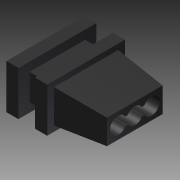
# Autodesk Inventor part: 276-2154
Saved by Autodesk Inventor 2013 (Build 170138000, 138)
## iProperties
Category: Sensors
Company: Autodesk Inc.
Created: 2012-03-30
Part Number: 276-2154
Document SubType Name: Modeling
Designer: Autodesk Inc.
Density: 0.93 g/cm^3
Material: Rubber
Catalog Web Link: http://www.vexrobotics.com/276-2154.html
Vendor: VEX
Mass: 0.0908272 g
Surface Area: 3.07194 cm^2
Volume: 0.0976637 cm^3
Author: Autodesk Inc.
Autodesk Inventor part; units mm, degrees
ref_plane "YZ Plane" through (0, 0, 0) normal (1, 0, 0) x (0, 1, 0)
ref_plane "XZ Plane" through (0, 0, 0) normal (0, 1, 0) x (-1, 0, 0)
ref_plane "XY Plane" through (0, 0, 0) normal (0, 0, 1) x (1, 0, 0)
sketch "Sketch1" plane through (0, 0, 0) normal (0, 0, 1) x (1, 0, 0)
  line L0 (0, 0) -> (7.0104, 0)
  line L1 (7.0104, 0) -> (7.0104, 3.9878)
  line L2 (7.0104, 3.9878) -> (0, 3.9878)
  line L3 (0, 3.9878) -> (0, 0)
  dimension "d0" = 7.0104
  dimension "d1" = 3.9878
  constraints: 8 end point, 2 parallel, 1 horizontal, 1 perpendicular
  measures "d0" distance of L2.end L1.end
  measures "d1" distance of L1.end L0.end
extrude "Extrusion1" add sketch "Sketch1" against normal blind 1.0922
sketch "Sketch2" plane through (0, 0, -1.0922) normal (0, 0, -1) x (-1, 0, 0)
  line L0 (-7.0104, 0) -> (-7.0104, 3.9878) projected
  line L1 (-7.0104, 3.9878) -> (0, 3.9878) projected
  line L2 (-6.0071, 0.8001) -> (-1.0033, 0.8001)
  line L3 (-1.0033, 0.8001) -> (-1.0033, 3.1877)
  line L4 (-1.0033, 3.1877) -> (-6.0071, 3.1877)
  line L5 (-6.0071, 3.1877) -> (-6.0071, 0.8001)
  point P0 (-3.5052, 3.1877)
  point P1 (-3.5052, 3.9878)
  point P2 (-6.0071, 1.9939)
  point P3 (-7.0104, 1.9939)
  dimension "d4" = 5.0038
  dimension "d5" = 2.3876
  constraints: 8 end point, 4 midpoint, 2 parallel, 1 horizontal, 1 horizontal alignment, 1 perpendicular, 1 vertical alignment
  measures "d4" distance of L3.end L4.end
  measures "d5" distance of L4.end L2.start
extrude "Extrusion2" add sketch "Sketch2" along normal blind 1.4986
pattern_linear "Rectangular Pattern1" count 2 spacing 2.5908 along (0, 0, -1) of "Extrusion1"
sketch "Sketch3" plane through (0, 0, 0) normal (0, 0, 1) x (1, 0, 0)
  line L0 (6.0071, 3.1877) -> (1.0033, 3.1877) projected
  line L1 (1.0033, 3.1877) -> (1.0033, 0.8001) projected
  line L2 (1.0033, 0.8001) -> (6.0071, 0.8001) projected
  line L3 (6.0071, 0.8001) -> (6.0071, 3.1877) projected
  line L4 (7.0104, 3.9878) -> (0, 3.9878) projected
  line L5 (0, 3.9878) -> (0, 0) projected
  line L6 (0.6096, 0.4953) -> (6.4008, 0.4953)
  line L7 (6.4008, 0.4953) -> (6.4008, 3.4925)
  line L8 (6.4008, 3.4925) -> (0.6096, 3.4925)
  line L9 (0.6096, 3.4925) -> (0.6096, 0.4953)
  point P0 (3.5052, 3.4925)
  point P1 (3.5052, 3.9878)
  point P2 (0.6096, 1.9939)
  point P3 (0, 1.9939)
  dimension "d14" = 5.7912
  dimension "d15" = 2.9972
  constraints: 8 end point, 4 midpoint, 2 parallel, 1 horizontal, 1 horizontal alignment, 1 perpendicular, 1 vertical alignment
  measures "d14" distance of L7.end L8.end
  measures "d15" distance of L8.end L6.start
sketch "Sketch3 outline for Extrusion3" plane through (0, 0, 0) normal (0, 0, 1) x (1, 0, 0)
  line L0 (0.6096, 3.4925) -> (0.6096, 0.4953)
  line L1 (6.4008, 3.4925) -> (0.6096, 3.4925)
  line L2 (6.4008, 0.4953) -> (6.4008, 3.4925)
  line L3 (0.6096, 0.4953) -> (6.4008, 0.4953)
extrude "Extrusion3" add sketch "Sketch3 outline for Extrusion3" along normal blind 4.3942 draft -5
sketch "Sketch4" plane through (0, 0, 4.3942) normal (0, 0, 1) x (1, 0, 0)
  line L0 (0.994043, 0.879743) -> (0.994043, 3.108057)
  line L1 (6.016357, 0.879743) -> (0.994043, 0.879743)
  line L2 (6.016357, 3.108057) -> (6.016357, 0.879743)
  line L3 (0.994043, 3.108057) -> (6.016357, 3.108057)
  line L4 (6.025892, 3.111592) -> (0.994043, 3.111592)
  line L5 (0.994043, 3.111592) -> (0.994043, 0.879743)
  line L6 (0.994043, 0.879743) -> (6.025892, 0.879743)
  line L7 (6.025892, 0.879743) -> (6.025892, 3.111592)
  line L8 (2.860448, 1.620667) -> (2.660448, 1.620667)
  arc A0 (2.660448, 2.370667) -> (2.660448, 1.620667) centre (2.010929, 1.995667) ccw
  line L9 (2.660448, 2.370667) -> (2.860448, 2.370667)
  arc A1 (4.159487, 2.370667) -> (2.860448, 2.370667) centre (3.509967, 1.995667) ccw
  line L10 (4.159487, 2.370667) -> (4.359487, 2.370667)
  arc A2 (4.359487, 1.620667) -> (4.359487, 2.370667) centre (5.009006, 1.995667) ccw
  line L11 (4.359487, 1.620667) -> (4.159487, 1.620667)
  arc A3 (2.860448, 1.620667) -> (4.159487, 1.620667) centre (3.509967, 1.995667) ccw
  point P0 (0, 0)
  constraints: 16 end point, 8 point on circle, 4 centre point
extrude "Extrusion4" cut sketch "Sketch4" against normal up to next contours L8 A0 L9 A1 L10 A2 L11 A3
body "Solid1"
